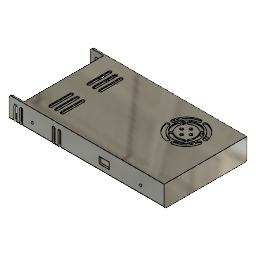
Mean Well LRS-350 Power Supply (Autodesk Fusion 360 design; units mm, degrees)
Autodesk Fusion 360 part; units mm, degrees
note: some values were not read from the file. Chosen so that the rebuilt part matches the saved one: which face or edge a step refers to; which pieces of a blend or face edit are solid.
sketch "Sketch1" plane through (0, 0, 0) normal (0, 0, 1) x (1, 0, 0)
  line L0 (0, 0) -> (215, 0)
  line L1 (215, 0) -> (215, 115)
  line L2 (215, 115) -> (0, 115)
  line L3 (0, 115) -> (0, 0)
  circle A0 centre (32.5, 32.5) radius 1.58
  circle A1 centre (32.5, 82.5) radius 1.58
  circle A2 centre (182.5, 82.5) radius 1.58
  circle A3 centre (182.5, 32.5) radius 1.58
  dimension "d1" = 215
  dimension "d2" = 115
  dimension "d3" = 3.16
  dimension "d4" = 3.16
  dimension "d5" = 3.16
  dimension "d6" = 3.16
  dimension "d7" = 32.5
  dimension "d8" = 32.5
  dimension "d9" = 32.5
  dimension "d10" = 32.5
  dimension "d11" = 150
  dimension "d12" = 150
  dimension "d13" = 50
  dimension "d14" = 32.5
  measures "d3" diameter of A0
  measures "d4" diameter of A1
  measures "d5" diameter of A2
  measures "d6" diameter of A3
extrude "Extrude1" add sketch "Sketch1" along normal blind 30
move_face "OffsetFaces1" offset 5 1 faces at (34.0721, 32.3427, 20)
delete_face "DeleteFace1" 1 faces at (31.7792, 81.094, 20)
delete_face "DeleteFace2" 1 faces at (183.3572, 83.8272, 20)
delete_face "DeleteFace3" 1 faces at (182.6965, 34.0677, 20)
extrude "Extrude2" cut sketch "Sketch1" along normal blind 6 contours A0 | A1 | A2 | A3
sketch "Sketch2" plane through (0, 0, 0) normal (0, -1, 0) x (1, 0, 0)
  line L0 (0, 0) -> (215, 0)
  line L1 (215, 0) -> (215, 30)
  line L2 (215, 30) -> (0, 30)
  line L3 (0, 30) -> (0, 0)
  circle A0 centre (32.5, 12.5) radius 1.58
  circle A1 centre (182.5, 12.5) radius 1.58
  dimension "d20" = 3.16
  dimension "d21" = 3.16
  dimension "d22" = 32.5
  dimension "d23" = 32.5
  dimension "d24" = 12.5
  dimension "d25" = 12.5
  measures "d20" diameter of A0
  measures "d21" diameter of A1
  measures "d22" distance of L0.start
  measures "d23" distance of L0.start
  measures "d24" distance of L0.start
  measures "d25" distance of L0.start
extrude "Extrude3" cut sketch "Sketch2" against normal blind 115 contours A0 | A1
sketch "Sketch3" plane through (0, 0, 30) normal (0, 0, 1) x (-1, 0, 0)
  line L0 (0, -115) -> (0, 0)
  line L1 (0, 0) -> (-215, 0)
  line L2 (-215, 0) -> (-215, -115)
  line L3 (-215, -115) -> (0, -115)
  line L4 (0, -112.5) -> (-18.7833, -112.5)
  line L5 (-18.7833, -112.5) -> (-18.7833, -2.5)
  line L6 (-18.7833, -2.5) -> (0, -2.5)
  line L7 (0, -2.5) -> (0, -112.5)
  dimension "d28" = 2.5
  dimension "d29" = 2.5
  measures "d28" distance of L0.end
  measures "d29" distance of L0.end
extrude "Extrude4" cut sketch "Sketch3" against normal blind 27.7 contours L0 L4 L5 L6 L7
sketch "Sketch4" plane through (18.7833, 0, 0) normal (-1, 0, 0) x (0, -1, 0)
  line L0 (-2.5, 30) -> (-112.5, 30)
  line L1 (-112.5, 30) -> (-112.5, 2.3)
  line L2 (-112.5, 2.3) -> (-2.5, 2.3)
  line L3 (-2.5, 2.3) -> (-2.5, 30)
  line L4 (-112.5, 2.3) -> (-2.5, 2.3)
  line L5 (-2.5, 2.3) -> (-2.5, 28.5)
  line L6 (-2.5, 28.5) -> (-112.5, 28.5)
  line L7 (-112.5, 28.5) -> (-112.5, 2.3)
  dimension "d32" = 26.2
  measures "d32" distance of origin
extrude "Extrude5" cut sketch "Sketch4" against normal blind 194.217 contours L1 L2 L3 L4 L5 L6 L7
sketch "Sketch5" plane through (0, 0, 30) normal (0, 0, 1) x (-1, 0, 0)
  line L0 (-18.7833, -2.5) -> (0, -2.5)
  line L1 (0, -2.5) -> (0, 0)
  line L2 (0, 0) -> (-215, 0)
  line L3 (-215, 0) -> (-215, -115)
  line L4 (-215, -115) -> (0, -115)
  line L5 (0, -115) -> (0, -112.5)
  line L6 (0, -112.5) -> (-18.7833, -112.5)
  line L7 (-18.7833, -112.5) -> (-18.7833, -2.5)
  line L8 (-215, 0) -> (-215, -115)
  line L9 (-215, -115) -> (0, -115)
  arc A0 (-163.1588, -102.9202) -> (-142.8798, -82.6412) centre (-167.5, -78.3) ccw
  arc A1 (-164.027, -97.9962) -> (-163.1588, -102.9202) centre (-163.5929, -100.4582) ccw
  arc A2 (-164.027, -97.9962) -> (-147.8038, -81.773) centre (-167.5, -78.3) ccw
  arc A3 (-142.8798, -82.6412) -> (-147.8038, -81.773) centre (-145.3418, -82.2071) ccw
  arc A4 (-163.5929, -100.4582) -> (-145.3418, -82.2071) centre (-167.5, -78.3) ccw construction
  line L10 (-167.5, -78.3) -> (-167.5, -115) construction
  line L11 (-167.5, -78.3) -> (-145, -78.3) construction
  arc A5 (-147.8038, -74.827) -> (-164.027, -58.6038) centre (-167.5, -78.3) ccw
  arc A6 (-142.8798, -73.9588) -> (-163.1588, -53.6798) centre (-167.5, -78.3) ccw
  arc A7 (-147.8038, -74.827) -> (-142.8798, -73.9588) centre (-145.3418, -74.3929) ccw
  arc A8 (-163.1588, -53.6798) -> (-164.027, -58.6038) centre (-163.5929, -56.1418) ccw
  arc A9 (-170.973, -58.6038) -> (-187.1962, -74.827) centre (-167.5, -78.3) ccw
  arc A10 (-171.8412, -53.6798) -> (-192.1202, -73.9588) centre (-167.5, -78.3) ccw
  arc A11 (-170.973, -58.6038) -> (-171.8412, -53.6798) centre (-171.4071, -56.1418) ccw
  arc A12 (-192.1202, -73.9588) -> (-187.1962, -74.827) centre (-189.6582, -74.3929) ccw
  arc A13 (-187.1962, -81.773) -> (-170.973, -97.9962) centre (-167.5, -78.3) ccw
  arc A14 (-192.1202, -82.6412) -> (-171.8412, -102.9202) centre (-167.5, -78.3) ccw
  arc A15 (-187.1962, -81.773) -> (-192.1202, -82.6412) centre (-189.6582, -82.2071) ccw
  arc A16 (-171.8412, -102.9202) -> (-170.973, -97.9962) centre (-171.4071, -100.4582) ccw
  arc A17 (-152.5773, -88.3655) -> (-152.5773, -68.2345) centre (-167.5, -78.3) ccw
  arc A18 (-156.7225, -85.5695) -> (-152.5773, -88.3655) centre (-154.6499, -86.9675) ccw
  arc A19 (-156.7225, -85.5695) -> (-156.7225, -71.0305) centre (-167.5, -78.3) ccw
  arc A20 (-152.5773, -68.2345) -> (-156.7225, -71.0305) centre (-154.6499, -69.6325) ccw
  arc A21 (-154.6499, -86.9675) -> (-154.6499, -69.6325) centre (-167.5, -78.3) ccw construction
  arc A22 (-160.2305, -67.5225) -> (-174.7695, -67.5225) centre (-167.5, -78.3) ccw
  arc A23 (-157.4345, -63.3773) -> (-177.5655, -63.3773) centre (-167.5, -78.3) ccw
  arc A24 (-160.2305, -67.5225) -> (-157.4345, -63.3773) centre (-158.8325, -65.4499) ccw
  arc A25 (-177.5655, -63.3773) -> (-174.7695, -67.5225) centre (-176.1675, -65.4499) ccw
  arc A26 (-178.2775, -71.0305) -> (-178.2775, -85.5695) centre (-167.5, -78.3) ccw
  arc A27 (-182.4227, -68.2345) -> (-182.4227, -88.3655) centre (-167.5, -78.3) ccw
  arc A28 (-178.2775, -71.0305) -> (-182.4227, -68.2345) centre (-180.3501, -69.6325) ccw
  arc A29 (-182.4227, -88.3655) -> (-178.2775, -85.5695) centre (-180.3501, -86.9675) ccw
  arc A30 (-174.7695, -89.0775) -> (-160.2305, -89.0775) centre (-167.5, -78.3) ccw
  arc A31 (-177.5655, -93.2227) -> (-157.4345, -93.2227) centre (-167.5, -78.3) ccw
  arc A32 (-174.7695, -89.0775) -> (-177.5655, -93.2227) centre (-176.1675, -91.1501) ccw
  arc A33 (-157.4345, -93.2227) -> (-160.2305, -89.0775) centre (-158.8325, -91.1501) ccw
  circle A34 centre (-167.5, -84.8) radius 2
  circle A35 centre (-161, -78.3) radius 2
  circle A36 centre (-167.5, -71.8) radius 2
  circle A37 centre (-174, -78.3) radius 2
  line L12 (-40.7833, -97) -> (-40.7833, -68)
  arc A38 (-40.7833, -68) -> (-44.7833, -68) centre (-42.7833, -68) ccw
  line L13 (-44.7833, -68) -> (-44.7833, -97)
  arc A39 (-44.7833, -97) -> (-40.7833, -97) centre (-42.7833, -97) ccw
  line L14 (-42.7833, -99) -> (-42.7833, -66) construction
  line L15 (-52.7833, -68) -> (-52.7833, -97)
  line L16 (-48.7833, -97) -> (-48.7833, -68)
  arc A40 (-48.7833, -68) -> (-52.7833, -68) centre (-50.7833, -68) ccw
  arc A41 (-52.7833, -97) -> (-48.7833, -97) centre (-50.7833, -97) ccw
  line L17 (-60.7833, -68) -> (-60.7833, -97)
  line L18 (-56.7833, -97) -> (-56.7833, -68)
  arc A42 (-56.7833, -68) -> (-60.7833, -68) centre (-58.7833, -68) ccw
  arc A43 (-60.7833, -97) -> (-56.7833, -97) centre (-58.7833, -97) ccw
  line L19 (-40.7833, -44) -> (-40.7833, -15)
  arc A44 (-40.7833, -15) -> (-44.7833, -15) centre (-42.7833, -15) ccw
  line L20 (-44.7833, -15) -> (-44.7833, -44)
  arc A45 (-44.7833, -44) -> (-40.7833, -44) centre (-42.7833, -44) ccw
  line L21 (-42.7833, -46) -> (-42.7833, -13) construction
  line L22 (-42.7833, -46) -> (-75.0949, -46) construction
  line L23 (-48.7833, -44) -> (-48.7833, -15)
  line L24 (-52.7833, -15) -> (-52.7833, -44)
  arc A46 (-52.7833, -44) -> (-48.7833, -44) centre (-50.7833, -44) ccw
  arc A47 (-48.7833, -15) -> (-52.7833, -15) centre (-50.7833, -15) ccw
  line L25 (-56.7833, -44) -> (-56.7833, -15)
  line L26 (-60.7833, -15) -> (-60.7833, -44)
  arc A48 (-60.7833, -44) -> (-56.7833, -44) centre (-58.7833, -44) ccw
  arc A49 (-56.7833, -15) -> (-60.7833, -15) centre (-58.7833, -15) ccw
  dimension "d43" = 47.5
  dimension "d44" = 36.7
  dimension "d46" = 5
  dimension "d51" = 360
  dimension "d52" = 15.5
  dimension "d53" = 70
  dimension "d54" = 68
  dimension "d55" = 5
  dimension "d56" = 10
  dimension "d58" = 360
  dimension "d59" = 25
  dimension "d60" = 4
  dimension "d61" = 6.5
  dimension "d63" = 360
  dimension "d64" = 33
  dimension "d65" = 4
  dimension "d66" = 22
  dimension "d67" = 18
  dimension "d70" = -8
  dimension "d71" = 0
  dimension "d72" = 33
  dimension "d73" = 90
  dimension "d74" = 4
  dimension "d75" = 15
  dimension "d78" = -8
  dimension "d79" = 0
  measures "d46" diameter of A3
  measures "d52" radius of A21
  measures "d53" angle of L1.end L2.start origin
  measures "d54" angle of L1.end L2.start origin
  measures "d56" angle of L1.end L2.start origin
  measures "d59" radius of A0
  measures "d60" diameter of A34
  measures "d65" diameter of A38
  measures "d66" distance of L7 L12
  measures "d72" distance of L1.end
  measures "d73" angle of L21 L22
  measures "d74" diameter of A44
extrude "Extrude6" cut sketch "Sketch5" against normal blind 7.617 contours A0 A1 A2 A3 | A5 A6 A7 A8 | A9 A10 A11 A12 | A13 A14 A15 A16 | A17 A18 A19 A20 | A22 A23 A24 A25 | A26 A27 A28 A29 | A30 A31 A32 A33 | A34 | A35 | A36 | A37 | L12 A38 L13 A39 | L15 L16 A40 A41 | L17 L18 A42 A43 | L19 A44 L20 A45 | L23 L24 A46 A47 | L25 L26 A48 A49
sketch "Sketch6" plane through (0, 0, 0) normal (0, -1, 0) x (1, 0, 0)
  circle A0 centre (32.5, 12.5) radius 1.58
  circle A1 centre (182.5, 12.5) radius 1.58
  line L0 (0, 0) -> (215, 0)
  line L1 (215, 0) -> (215, 30)
  line L2 (215, 30) -> (0, 30)
  line L3 (0, 30) -> (0, 0)
  line L4 (7, 21) -> (7, 0)
  arc A2 (7, 0) -> (11, 0) centre (9, 0) ccw
  line L5 (11, 0) -> (11, 21)
  arc A3 (11, 21) -> (7, 21) centre (9, 21) ccw
  line L6 (9, 23) -> (9, -2) construction
  line L7 (9, 23) -> (30.2877, 23) construction
  line L8 (15, 21) -> (15, 0)
  line L9 (19, 0) -> (19, 21)
  arc A4 (19, 21) -> (15, 21) centre (17, 21) ccw
  arc A5 (15, 0) -> (19, 0) centre (17, 0) ccw
  dimension "d80" = 25
  dimension "d81" = 90
  dimension "d82" = 4
  dimension "d83" = 7
  dimension "d84" = 9
  dimension "d87" = 8
  dimension "d88" = 0
  measures "d81" angle of L6 L7
  measures "d82" diameter of A2
  measures "d83" distance of L3 L4
extrude "Extrude7" cut sketch "Sketch6" against normal up to surface (2.5 mm away) contours L0 L4 L5 A3 | L0 L8 L9 A4
ref_plane "WorkPlane1" through (107.5, 57.5, 15) normal (0, -1, 0) x (1, 0, 0)
mirror "Mirror1" about plane through (107.5, 57.5, 15) normal (0, -1, 0) of "Extrude7"
sketch "Sketch7" plane through (0, 0, 0) normal (0, -1, 0) x (1, 0, 0)
  circle A0 centre (182.5, 12.5) radius 1.58
  circle A1 centre (32.5, 12.5) radius 1.58
  line L0 (0, 30) -> (0, 0)
  line L1 (0, 0) -> (7, 0)
  line L2 (7, 0) -> (7, 21)
  arc A2 (11, 21) -> (7, 21) centre (9, 21) ccw
  line L3 (11, 21) -> (11, 0)
  line L4 (11, 0) -> (15, 0)
  line L5 (15, 0) -> (15, 21)
  arc A3 (19, 21) -> (15, 21) centre (17, 21) ccw
  line L6 (19, 21) -> (19, 0)
  line L7 (19, 0) -> (215, 0)
  line L8 (215, 0) -> (215, 30)
  line L9 (215, 30) -> (0, 30)
  arc A4 (11, 21) -> (7, 21) centre (9, 21) ccw
  arc A5 (19, 21) -> (15, 21) centre (17, 21) ccw
  line L10 (19, 21) -> (19, 0)
  line L11 (15, 0) -> (15, 21)
  line L12 (11, 21) -> (11, 0)
  line L13 (7, 0) -> (7, 21)
  line L14 (60, 21) -> (60, 0)
  arc A6 (60, 0) -> (64, 0) centre (62, 0) ccw
  line L15 (64, 0) -> (64, 21)
  arc A7 (64, 21) -> (60, 21) centre (62, 21) ccw
  line L16 (62, 23) -> (62, -2) construction
  line L17 (62, 23) -> (87, 23) construction
  line L18 (72, 0) -> (72, 21)
  line L19 (68, 21) -> (68, 0)
  arc A8 (68, 0) -> (72, 0) centre (70, 0) ccw
  arc A9 (72, 21) -> (68, 21) centre (70, 21) ccw
  dimension "d92" = 25
  dimension "d93" = 90
  dimension "d94" = 4
  dimension "d95" = 60
  dimension "d98" = 8
  dimension "d99" = 0
  measures "d92" distance of L0.end
  measures "d93" angle of L16 L17
  measures "d94" diameter of A6
  measures "d95" distance of L0 L14
extrude "Extrude8" cut sketch "Sketch7" against normal up to surface (2.5 mm away) contours L7 L18 L19 A9 | L7 L14 L15 A7
sketch "Sketch8" plane through (0, 0, 0) normal (0, 0, -1) x (1, 0, 0)
  line L0 (72, 0) -> (72, -2.5)
  line L1 (72, -2.5) -> (68, -2.5)
  line L2 (68, -2.5) -> (68, 0)
  line L3 (68, 0) -> (64, 0)
  line L4 (64, 0) -> (64, -2.5)
  line L5 (64, -2.5) -> (60, -2.5)
  line L6 (60, -2.5) -> (60, 0)
  line L7 (60, 0) -> (19, 0)
  line L8 (19, 0) -> (19, -2.5)
  line L9 (19, -2.5) -> (15, -2.5)
  line L10 (15, -2.5) -> (15, 0)
  line L11 (15, 0) -> (11, 0)
  line L12 (11, 0) -> (11, -2.5)
  line L13 (11, -2.5) -> (7, -2.5)
  line L14 (7, -2.5) -> (7, 0)
  line L15 (7, 0) -> (0, 0)
  line L16 (0, 0) -> (0, -115)
  line L17 (0, -115) -> (7, -115)
  line L18 (7, -115) -> (7, -112.5)
  line L19 (7, -112.5) -> (11, -112.5)
  line L20 (11, -112.5) -> (11, -115)
  line L21 (11, -115) -> (15, -115)
  line L22 (15, -115) -> (15, -112.5)
  line L23 (15, -112.5) -> (19, -112.5)
  line L24 (19, -112.5) -> (19, -115)
  line L25 (19, -115) -> (215, -115)
  line L26 (215, -115) -> (215, 0)
  line L27 (215, 0) -> (72, 0)
  circle A0 centre (182.5, -82.5) radius 1.58
  circle A1 centre (32.5, -32.5) radius 1.58
  circle A2 centre (182.5, -32.5) radius 1.58
  circle A3 centre (32.5, -82.5) radius 1.58
  line L28 (7, 0) -> (7, -4)
  arc A4 (7, -4) -> (11, -4) centre (9, -4) ccw
  line L29 (11, -4) -> (11, 0)
  arc A5 (11, 0) -> (7, 0) centre (9, 0) ccw
  line L30 (9, 0) -> (9, -4) construction
  line L31 (7, 0) -> (11, 0)
  line L32 (9, 0) -> (13, 0) construction
  arc A6 (15, -4) -> (19, -4) centre (17, -4) ccw
  line L33 (19, -4) -> (19, 0)
  arc A7 (19, 0) -> (15, 0) centre (17, 0) ccw
  line L34 (15, 0) -> (15, -4)
  arc A8 (72, 0) -> (68, 0) centre (70, 0) ccw
  line L35 (72, 0) -> (72, -2.5)
  line L36 (68, -2.5) -> (68, 0)
  line L37 (68, 0) -> (64, 0)
  line L38 (64, 0) -> (64, -2.5)
  arc A9 (68, -4) -> (72, -4) centre (70, -4) ccw
  line L39 (64, -2.5) -> (60, -2.5)
  arc A10 (64, 0) -> (60, 0) centre (62, 0) ccw
  line L40 (72, -2.5) -> (68, -2.5)
  line L41 (62, 0) -> (66, 0) construction
  line L42 (68, 0) -> (68, -4)
  line L43 (72, -4) -> (72, 0)
  line L44 (64, -4) -> (64, 0)
  line L45 (62, 0) -> (62, -4) construction
  line L46 (60, -2.5) -> (60, 0)
  arc A11 (60, -4) -> (64, -4) centre (62, -4) ccw
  line L47 (60, 0) -> (60, -4)
  line L48 (60, 0) -> (64, 0)
  arc A12 (19, -110) -> (15, -110) centre (17, -110) ccw
  line L49 (11, -110) -> (11, -112.5)
  line L50 (7, -112.5) -> (7, -110)
  line L51 (11, -112.5) -> (7, -112.5)
  arc A13 (15, -114) -> (19, -114) centre (17, -114) ccw
  arc A14 (11, -110) -> (7, -110) centre (9, -110) ccw
  line L52 (15, -110) -> (11, -110)
  line L53 (15, -112.5) -> (15, -110)
  line L54 (9, -110) -> (13, -110) construction
  line L55 (19, -112.5) -> (15, -112.5)
  line L56 (19, -110) -> (19, -112.5)
  line L57 (9, -110) -> (9, -114) construction
  line L58 (7, -110) -> (11, -110)
  line L59 (11, -114) -> (11, -110)
  line L60 (15, -110) -> (15, -114)
  arc A15 (7, -114) -> (11, -114) centre (9, -114) ccw
  line L61 (19, -114) -> (19, -110)
  line L62 (7, -110) -> (7, -114)
  dimension "d102" = 4
  dimension "d103" = 90
  dimension "d104" = 4
  dimension "d107" = 8
  dimension "d108" = 0
  dimension "d111" = 53
  dimension "d112" = 0
  dimension "d115" = 0
  dimension "d116" = -110
  measures "d103" angle of L30 L32
  measures "d104" diameter of A4
extrude "Extrude9" cut sketch "Sketch8" against normal up to surface (2.3 mm away) contours L0 L1 L2 A8 L35 L36 L40 L42 L43 | L1 A9 L40 L42 L43 | A10 L48 | L4 L5 L6 L38 L39 L44 L46 L47 L48 | L5 L39 L44 A11 L47 | L22 L23 L24 A13 L55 L60 L61 | L8 L9 L10 L33 A7 L34 | L23 A12 L53 L55 L56 L60 L61 | L9 A6 L33 L34 | A5 L31 | L12 L13 L14 L28 L29 L31 | L13 L28 A4 L29 | A14 L58 | L19 L49 L50 L51 L58 L59 L62 | L18 L19 L20 L51 L59 A15 L62
sketch "Sketch9" plane through (0, 0, 0) normal (0, -1, 0) x (1, 0, 0)
  line L0 (72, 21) -> (72, 0)
  line L1 (72, 0) -> (215, 0)
  line L2 (215, 0) -> (215, 30)
  line L3 (215, 30) -> (0, 30)
  line L4 (0, 30) -> (0, 0)
  line L5 (0, 0) -> (7, 0)
  line L6 (7, 0) -> (7, 21)
  arc A0 (11, 21) -> (7, 21) centre (9, 21) ccw
  line L7 (11, 21) -> (11, 0)
  line L8 (11, 0) -> (15, 0)
  line L9 (15, 0) -> (15, 21)
  arc A1 (19, 21) -> (15, 21) centre (17, 21) ccw
  line L10 (19, 21) -> (19, 0)
  line L11 (19, 0) -> (60, 0)
  line L12 (60, 0) -> (60, 21)
  arc A2 (64, 21) -> (60, 21) centre (62, 21) ccw
  line L13 (64, 21) -> (64, 0)
  line L14 (64, 0) -> (68, 0)
  line L15 (68, 0) -> (68, 21)
  arc A3 (72, 21) -> (68, 21) centre (70, 21) ccw
  circle A4 centre (182.5, 12.5) radius 1.58
  circle A5 centre (32.5, 12.5) radius 1.58
  line L16 (125, 18.5) -> (139, 18.5)
  line L17 (139, 18.5) -> (139, 9.5)
  line L18 (139, 9.5) -> (125, 9.5)
  line L19 (125, 9.5) -> (125, 18.5)
  dimension "d119" = 14
  dimension "d120" = 9
  dimension "d121" = 76
  dimension "d122" = 9.5
  measures "d121" distance of L2 L17
  measures "d122" distance of L1 L18
extrude "Extrude10" cut sketch "Sketch9" against normal up to surface (2.5 mm away) contours L16 L17 L18 L19
fillet "Fillet1" radius 3 2 edges at (0, 1.25, 30) (0, 113.75, 30)
fillet "Fillet2" radius 3 16 edges at (3.5, 0, 0) (143.5, 0, 0) (13, 0, 0) (66, 0, 0) (39.5, 0, 0) (3.5, 115, 0) (7, 2, 0) (11, 2, 0) (15, 2, 0) (19, 2, 0) (60, 2, 0) (64, 2, 0) (68, 2, 0) (72, 2, 0) (117, 115, 0) (13, 115, 0)
fillet "Fillet3" radius 1.5 8 edges at (3.5, 112.5, 2.3) (116.0002, 112.5, 2.3) (13, 112.5, 2.3) (142.5002, 2.5, 2.3) (66, 2.5, 2.3) (39.5, 2.5, 2.3) (13, 2.5, 2.3) (3.5, 2.5, 2.3)
equation "d30 = -30.00 mm + 2.3 mm"
equation "d32 = 27.700 mm - 1.5 mm"
